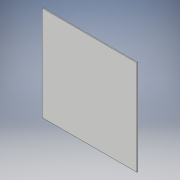
# Autodesk Inventor part: screen
Saved by Autodesk Inventor 2019 (Build 230136000, 136)
## iProperties
Created: 2018-07-11
Part Number: screen
Material: Generic
Document SubType Name: Modeling
Designer: User
Density: 1 g/cm^3
Appearance: Default
Author: User
Autodesk Inventor part; units mm, degrees
ref_plane "YZ Plane" through (0, 0, 0) normal (1, 0, 0) x (0, 1, 0)
ref_plane "XZ Plane" through (0, 0, 0) normal (0, 1, 0) x (-1, 0, 0)
ref_plane "XY Plane" through (0, 0, 0) normal (0, 0, 1) x (1, 0, 0)
sketch "Sketch1" plane through (0, 0, 0) normal (0, 0, 1) x (1, 0, 0)
  line L0 (-139.7, -139.7) -> (139.7, -139.7)
  line L1 (139.7, -139.7) -> (139.7, 139.7)
  line L2 (139.7, 139.7) -> (-139.7, 139.7)
  line L3 (-139.7, 139.7) -> (-139.7, -139.7)
  line L4 (-139.7, -139.7) -> (139.7, 139.7) construction
  line L5 (139.7, -139.7) -> (-139.7, 139.7) construction
  point P0 (0, 0)
  dimension "d0" = 279.4
  constraints: 12 end point, 2 midpoint, 2 parallel, 2 perpendicular, 1 horizontal
  measures "d0" distance of L1.end L2.end
extrude "Extrusion1" add sketch "Sketch1" along normal blind 2.54
body "Solid1"
